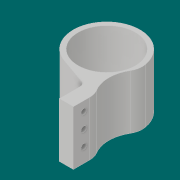
# Autodesk Inventor part: MotorMountA
Saved by Autodesk Inventor 2018 (Build 220112000, 112)
## iProperties
Created: 2018-01-25
Part Number: MotorMountA
Material: Generic
Document SubType Name: Modeling
Designer: Mira
Density: 1 g/cm^3
Appearance: Default
Author: Mira
Autodesk Inventor part; units mm, degrees
ref_plane "YZ Plane" through (0, 0, 0) normal (1, 0, 0) x (0, 1, 0)
ref_plane "XZ Plane" through (0, 0, 0) normal (0, 1, 0) x (-1, 0, 0)
ref_plane "XY Plane" through (0, 0, 0) normal (0, 0, 1) x (1, 0, 0)
sketch "Sketch1" plane through (0, 0, 0) normal (0, 1, 0) x (-1, 0, 0)
  arc A0 (-22.225, 0) -> (7.3478, 20.9752) centre (0, 0) ccw
  line L0 (-22.225, 0) -> (-12.7, 0)
  line L1 (-12.7, 44.45) -> (-22.225, 44.45)
  line L2 (-22.225, 44.45) -> (-22.225, 0)
  line L3 (39.7917, 0) -> (-48.1139, 0) construction
  line L4 (-10.5747, 27.2537) -> (7.3478, 20.9752)
  line L5 (-12.7, 30.2501) -> (-12.7, 44.45)
  arc A1 (-12.7, 30.2501) -> (-10.5747, 27.2537) centre (-9.525, 30.2501) ccw
  dimension "d0" = 44.45
  dimension "d3" = 9.525
  dimension "d4" = 44.45
  dimension "d5" = 3.175
  constraints: 12 end point, 4 point on circle, 3 horizontal, 3 tangent, 2 centre point, 2 parallel, 1 coincident, 1 perpendicular, 1 point on line, 1 other
  measures "d0" diameter of A0
  measures "d3" distance of L1.start L1.end
  measures "d4" distance of L0.start L1.end
  measures "d5" radius of A1
extrude "Extrusion1" add sketch "Sketch1" along normal blind 25.4
sketch "Sketch2" plane through (0, 25.4, 0) normal (0, 1, 0) x (1, 0, 0)
  circle A0 centre (0, 0) radius 19.05
  dimension "d8" = 38.1
  constraints: 1 centre point, 1 coincident
  measures "d8" diameter of A0
extrude "Extrusion2" cut sketch "Sketch2" against normal blind 20.32
sketch "Sketch3" plane through (0, 5.08, 0) normal (0, 1, 0) x (1, 0, 0)
  circle A0 centre (0, 15.875) radius 1.9844
  circle A1 centre (0, 0) radius 19.05 projected
  circle A2 centre (-13.7482, 7.9375) radius 1.9844
  circle A3 centre (-13.7482, -7.9375) radius 1.9844
  circle A4 centre (0, -15.875) radius 1.9844
  circle A5 centre (13.7482, -7.9375) radius 1.9844
  circle A6 centre (13.7482, 7.9375) radius 1.9844
  circle A7 centre (0, 0) radius 13.4938
  point P0 (0, 0)
  point P1 (0, 19.05)
  dimension "d11" = 3.9688
  dimension "d12" = 3.175
  dimension "d15" = 360
  dimension "d17" = 5.5563
  constraints: 7 centre point, 1 coincident, 1 vertical alignment, 14 other
  measures "d11" diameter of A0
  measures "d12" distance of A0.centre point (0, 19.05)
extrude "Extrusion3" cut sketch "Sketch3" against normal up to next contours A0 | A2 | A3 | A4 | A5 | A6 | A7
sketch "Sketch5" plane through (0, 25.4, 0) normal (0, 1, 0) x (1, 0, 0)
  circle A0 centre (0, 0) radius 19.05 projected
  line L0 (12.7, -44.45) -> (22.225, -44.45) projected
  line L1 (22.225, -44.45) -> (22.225, 0) projected
  arc A1 (22.225, 0) -> (-7.3478, -20.9752) centre (0, 0) ccw projected
  line L2 (-7.3478, -20.9752) -> (10.5747, -27.2537) projected
  arc A2 (12.7, -30.2501) -> (10.5747, -27.2537) centre (9.525, -30.2501) ccw projected
  line L3 (12.7, -30.2501) -> (12.7, -44.45) projected
extrude "Extrusion5" add sketch "Sketch5" along normal blind 7.62
sketch "Sketch4" plane through (12.7, 0, 30.2501) normal (-1, 0, 0) x (0, 0, 1)
  circle A0 centre (7.0999, 26.67) radius 1.8034
  line L0 (0, 0) -> (0, 25.4) construction
  line L1 (0, 24.4432) -> (14.1999, 24.4432) construction
  line L2 (14.1999, 24.4432) -> (7.0999, 24.4432) construction
  line L3 (7.0999, 24.4432) -> (7.0999, 0) construction
  line L4 (14.1999, 0) -> (-30.2501, 0) construction
  circle A1 centre (7.0999, 16.51) radius 1.8034
  circle A2 centre (7.0999, 6.35) radius 1.8034
  line L5 (14.1999, 0) -> (14.1999, 33.02) projected
  line L6 (14.1999, 16.51) -> (0, 16.51) construction
  dimension "d20" = 3.6068
  dimension "d21" = 3.6068
  dimension "d22" = 3.6068
  dimension "d23" = 10.16
  dimension "d24" = 10.16
  constraints: 8 end point, 6 point on line, 3 centre point, 3 midpoint, 2 perpendicular, 1 horizontal
  measures "d20" diameter of A0
  measures "d21" diameter of A1
  measures "d22" diameter of A2
  measures "d23" distance of A0.centre A1.centre
  measures "d24" distance of A2.centre A1.centre
extrude "Extrusion4" cut sketch "Sketch4" against normal up to next
sketch "Sketch6" plane through (0, 33.02, 0) normal (0, 1, 0) x (1, 0, 0)
  line L0 (22.225, -44.45) -> (22.225, 0) projected
  line L1 (22.225, -22.225) -> (22.225, -4.0892)
  line L2 (22.225, -44.45) -> (22.225, 0) projected
  arc A0 (22.225, -2.0148) -> (22.225, -29.6579) centre (39.2288, -15.8363) ccw
  line L3 (22.225, -29.6579) -> (22.225, -2.0148)
  point P0 (0, 0)
  constraints: 4 end point, 3 point on line, 2 collinear, 2 point on circle, 1 centre point, 1 midpoint
extrude "Extrusion6" cut sketch "Sketch6" against normal up to next
fillet "Fillet1" radius 12.7 2 edges at (22.225, 16.51, 29.6579) (22.225, 16.51, 2.0148)
sketch "Sketch7" plane through (0, 0, 0) normal (0, -1, 0) x (1, 0, 0)
  arc A0 (21.8765, -3.9203) -> (20.3293, 4.747) centre (9.3757, -1.6801) ccw projected
  arc A1 (20.4239, 27.0852) -> (20.3293, 4.747) centre (39.2288, 15.8363) ccw projected
  arc A2 (20.4239, 27.0852) -> (22.225, 33.6048) centre (9.525, 33.6048) ccw projected
  line L0 (22.225, 44.45) -> (22.225, 33.6048) projected
  line L1 (12.7, 44.45) -> (22.225, 44.45) projected
  line L2 (12.7, 30.2501) -> (12.7, 44.45) projected
  arc A3 (10.5747, 27.2537) -> (12.7, 30.2501) centre (9.525, 30.2501) ccw projected
  line L3 (-7.3478, 20.9752) -> (10.5747, 27.2537) projected
  arc A4 (-7.3478, 20.9752) -> (21.8765, -3.9203) centre (0, 0) ccw projected
  circle A5 centre (0, 0) radius 13.4938 projected
  circle A6 centre (13.7482, 7.9375) radius 1.9844 projected
  circle A7 centre (-13.7482, 7.9375) radius 1.9844 projected
  circle A8 centre (0, -15.875) radius 1.9844 projected
  circle A9 centre (-13.7482, -7.9375) radius 1.9844 projected
  circle A10 centre (0, 15.875) radius 1.9844 projected
  circle A11 centre (13.7482, -7.9375) radius 1.9844 projected
extrude "Extrusion7" add sketch "Sketch7" along normal blind 3.175
body "Solid1"
